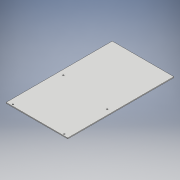
# Autodesk Inventor part: trunk
Saved by Autodesk Inventor 2018 (Build 220112000, 112)
## iProperties
Created: 2018-06-06
Part Number: trunk
Material: Generic
Document SubType Name: Modeling
Designer: John Viljoen
Density: 1 g/cm^3
Appearance: Default
Author: John Viljoen
Autodesk Inventor part; units mm, degrees
ref_plane "YZ Plane" through (0, 0, 0) normal (1, 0, 0) x (0, 1, 0)
ref_plane "XZ Plane" through (0, 0, 0) normal (0, 1, 0) x (-1, 0, 0)
ref_plane "XY Plane" through (0, 0, 0) normal (0, 0, 1) x (1, 0, 0)
sketch "Sketch1" plane through (0, 0, 0) normal (0, 0, 1) x (1, 0, 0)
  line L0 (0, 0) -> (189.177, 0)
  line L1 (189.177, 0) -> (189.177, 325.825)
  line L2 (189.177, 325.825) -> (0, 325.825)
  line L3 (0, 325.825) -> (0, 0)
  dimension "d0" = 189.177
  dimension "d1" = 325.825
  constraints: 8 end point, 2 parallel, 1 horizontal, 1 perpendicular
  measures "d0" distance of L2.end L1.end
  measures "d1" distance of L1.end L0.end
extrude "Extrusion1" add sketch "Sketch1" along normal blind 2.6
sketch "Sketch2" plane through (0, 0, 2.6) normal (0, 0, 1) x (1, 0, 0)
  line L0 (0, 170) -> (0, 0)
  line L1 (0, 170) -> (0, 159.84) construction
  line L2 (0, 159.84) -> (6.35, 159.84) construction
  line L3 (6.35, 170) -> (163.83, 170) construction
  line L4 (163.83, 170) -> (163.83, 136.98) construction
  line L5 (6.35, 159.84) -> (6.35, 4.9) construction
  line L6 (6.35, 4.9) -> (163.83, 4.9) construction
  line L7 (6.35, 159.84) -> (15.9385, 159.84) construction
  line L8 (15.9385, 159.84) -> (15.9385, 4.9) construction
  line L9 (163.83, 136.98) -> (173.4185, 136.98) construction
  line L10 (173.4185, 136.98) -> (173.4185, 4.9) construction
  circle A0 centre (15.9385, 4.9) radius 1.98
  circle A1 centre (173.4185, 4.9) radius 1.98
  circle A2 centre (15.9385, 159.84) radius 1.98
  circle A3 centre (173.4185, 136.98) radius 1.98
  dimension "d4" = 10.16
  dimension "d6" = 157.48
  dimension "d7" = 33.02
  dimension "d8" = 154.94
  dimension "d13" = 9.5885
  dimension "d14" = 9.5885
  dimension "d15" = 3.96
  dimension "d16" = 3.96
  dimension "d17" = 3.96
  dimension "d18" = 3.96
  constraints: 22 end point, 6 coincident, 5 perpendicular, 4 centre point, 2 horizontal, 2 point on line, 1 vertical
  measures "d4" distance of L0.start L1.end
  measures "d6" distance of L3.start L3.end
  measures "d7" distance of L3.end L4.end
  measures "d8" distance of L2.end L5.end
  measures "d13" distance of L7.start L7.end
  measures "d14" distance of L9.start L9.end
  measures "d15" diameter of A0
  measures "d16" diameter of A1
  measures "d17" diameter of A2
  measures "d18" diameter of A3
extrude "Extrusion2" cut sketch "Sketch2" against normal blind 5
body "Solid1"
